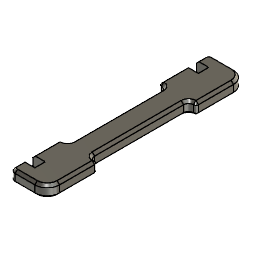
Rubber Band Tensioner (Autodesk Fusion 360 design; units mm, degrees)
Autodesk Fusion 360 part; units mm, degrees
sketch "Sketch1" plane through (0, 0, 0) normal (0, 0, 1) x (1, 0, 0)
  line L0 (7.5, -40.2) -> (-7.5, -40.2)
  line L1 (-7.5, -40.2) -> (-7.5, 40.2)
  line L2 (-7.5, 40.2) -> (7.5, 40.2)
  line L3 (7.5, 40.2) -> (7.5, -40.2)
  line L4 (7.5, -40.2) -> (-7.5, 40.2) construction
  line L5 (-7.5, -40.2) -> (7.5, 40.2) construction
  line L6 (-7.5, 35.2) -> (-2.5, 35.2)
  line L7 (-2.5, 35.2) -> (-2.5, 31)
  line L8 (-2.5, 31) -> (-7.5, 31)
  line L9 (-7.5, 31) -> (-7.5, 35.2)
  line L10 (-7.5, -31) -> (-2.5, -31)
  line L11 (-2.5, -31) -> (-2.5, -35.2)
  line L12 (-2.5, -35.2) -> (-7.5, -35.2)
  line L13 (-7.5, -35.2) -> (-7.5, -31)
  line L14 (0, 1.75) -> (0, 22.5)
  line L15 (-7.5, 20) -> (-4.5, 20)
  line L16 (-4.5, 20) -> (-4.5, -20)
  line L17 (-4.5, -20) -> (-7.5, -20)
  line L18 (-7.5, -20) -> (-7.5, 20)
  line L19 (7.5, -20) -> (4.5, -20)
  line L20 (4.5, -20) -> (4.5, 20)
  line L21 (4.5, 20) -> (7.5, 20)
  line L22 (7.5, 20) -> (7.5, -20)
  dimension "d1" = 80.4
  dimension "d2" = 15
  dimension "d3" = 5
  dimension "d4" = 4.2
  dimension "d5" = 5
  dimension "d6" = 4.2
  dimension "d7" = 5
  dimension "d8" = 5
  dimension "d26" = 15
  dimension "d27" = 40.2
  dimension "d28" = 3
  dimension "d29" = 40
  dimension "d30" = 20
  dimension "d31" = 40
  dimension "d32" = 3
  dimension "d33" = 20
  constraint horizontal L0
  constraint perpendicular L0 L1
  constraint parallel L0 L2
  constraint horizontal L6
  constraint vertical L7
  constraint horizontal L8
  constraint vertical L9
  constraint coincident L1 L6.start
  constraint horizontal L10
  constraint vertical L11
  constraint horizontal L12
  constraint vertical L13
  constraint coincident L1 L10.start
  constraint symmetric L4 L5 L14
  constraint horizontal L15
  constraint vertical L16
  constraint horizontal L17
  constraint vertical L18
  constraint coincident L1 L15.start
  constraint horizontal L19
  constraint vertical L20
  constraint horizontal L21
  constraint vertical L22
  constraint coincident L3 L19.start
  measures "d1" distance of L0.end L1.end
  measures "d2" distance of L0.start L0.end
  measures "d3" distance of L6.start L6.end
  measures "d4" distance of L6.start L8.end
  measures "d5" distance of L10.start L10.end
  measures "d6" distance of L10.start L12.end
  measures "d7" distance of L0 L12
  measures "d8" distance of L2 L6
  measures "d26" distance of L1.end L2.end
  measures "d27" distance of origin L0
  measures "d28" distance of L15.start L15.end
  measures "d29" distance of L15.end L16.end
  measures "d30" distance of origin L15
  measures "d31" distance of L19.end L20.end
  measures "d32" distance of L19.start L19.end
  measures "d33" distance of origin L21
extrude "Extrude1" add sketch "Sketch1" along normal blind 4.8 contours L0 L1 L2 L3 L6 L7 L8 L10 L11 L12 L15 L16 L17 L19 L20 L21
fillet "Fillet1" radius 5 2 edges at (7.5, 40.2, 2.4) (7.5, -40.2, 2.4)
fillet "Fillet1" radius 2 6 edges at (-7.5, 40.2, 2.4) (-7.5, -40.2, 2.4) (-4.5, 20, 2.4) (4.5, 20, 2.4) (4.5, -20, 2.4) (-4.5, -20, 2.4)
fillet "Fillet1" radius 1 4 edges at (-7.5, 20, 2.4) (7.5, 20, 2.4) (-7.5, -20, 2.4) (7.5, -20, 2.4)
chamfer "Chamfer1" distance 1 angle 45 44 edges at (7.5, 28.1, 4.8) (7.2071, 20.2929, 4.8) (5.0858, 19.4142, 4.8) (4.5, 0, 4.8) (5.0858, -19.4142, 4.8) (7.2071, -20.2929, 4.8) (7.5, -28.1, 4.8) (6.0355, -38.7355, 4.8) (-1.5, -40.2, 4.8) (-6.9142, -39.6142, 4.8) (-7.5, -36.7, 4.8) (-7.5, 36.7, 4.8) (-6.9142, 39.6142, 4.8) (-1.5, 40.2, 4.8) (6.0355, 38.7355, 4.8) (7.5, -28.1, 0) (7.2071, -20.2929, 0) (5.0858, -19.4142, 0) (4.5, 0, 0) (5.0858, 19.4142, 0) (7.2071, 20.2929, 0) (7.5, 28.1, 0) (6.0355, 38.7355, 0) (-1.5, 40.2, 0) (-6.9142, 39.6142, 0) (-7.5, 36.7, 0) (-7.5, -36.7, 0) (-6.9142, -39.6142, 0) (-1.5, -40.2, 0) (6.0355, -38.7355, 0) (-7.5, -26, 0) (-7.2071, -20.2929, 0) (-5.0858, -19.4142, 0) (-4.5, 0, 0) (-5.0858, 19.4142, 0) (-7.2071, 20.2929, 0) (-7.5, 26, 0) (-7.5, 26, 4.8) (-7.2071, 20.2929, 4.8) (-5.0858, 19.4142, 4.8) (-4.5, 0, 4.8) (-5.0858, -19.4142, 4.8) (-7.2071, -20.2929, 4.8) (-7.5, -26, 4.8)
equation "d27 = d1 / 2"
equation "d30 = d29 / 2"
equation "d33 = d31 / 2"
